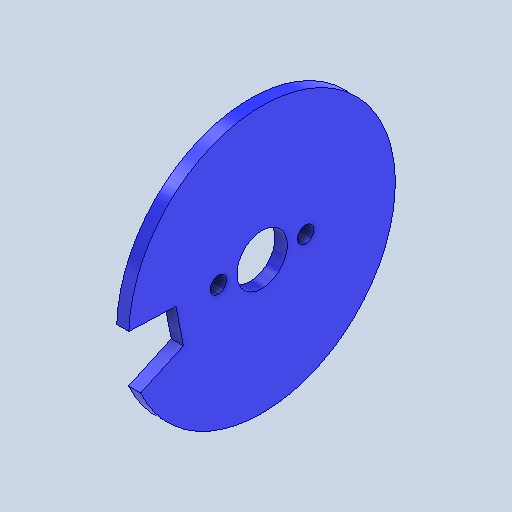
# Autodesk Inventor part: belt_liner_v2_3DP_P-1-F
Saved by Autodesk Inventor 2025.2 (Build 292293000, 293)
## iProperties
Created: 2025-01-13
Part Number: belt_liner_v2_3DP_P-1-F
Material: ABS プラスチック
Document SubType Name: Modeling
Designer: haruy
Density: 1.06 g/cm^3
Appearance: 青 - 壁塗料 - 光沢
Author: haruy
Autodesk Inventor part; units mm, degrees
ref_plane "YZ Plane" through (0, 0, 0) normal (1, 0, 0) x (0, 1, 0)
ref_plane "XZ Plane" through (0, 0, 0) normal (0, 1, 0) x (-1, 0, 0)
ref_plane "XY Plane" through (0, 0, 0) normal (0, 0, 1) x (1, 0, 0)
sketch "スケッチ1" plane through (0, 0, 0) normal (1, 0, 0) x (0, 1, 0)
  arc A0 (-5.655, 32.8818) -> (6.5548, 35.3105) centre (5.6756, 7.8246) ccw
  circle A1 centre (5.6756, -1.1754) radius 1.7
  circle A2 centre (5.6756, 16.8246) radius 1.7
  circle A3 centre (5.6756, 7.8246) radius 5.2
  line L0 (-1.6304, 24.0509) -> (-5.655, 32.8818)
  line L1 (6.5548, 35.3105) -> (6.2159, 25.6116)
  line L2 (6.2159, 25.6116) -> (-1.6304, 24.0509)
  point P0 (0, 0)
  constraints: 6 end point, 4 centre point, 2 point on circle
extrude "押し出し1" add sketch "スケッチ1" along normal blind 2.5
